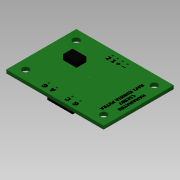
# Autodesk Inventor part: UVTRON
Saved by Autodesk Inventor 2015 SP1 (Build 190203100, 203)
## iProperties
Created: 2015-01-27
Part Number: UVTRON
Material: Generic
Document SubType Name: Modeling
Designer: Rafi Kurnia Putra
Density: 1 g/cm^3
Appearance: Smooth - Dark Forest Green
Mass: 4.62788 g
Surface Area: 45.4293 cm^2
Volume: 4.62788 cm^3
Author: Rafi Kurnia Putra
Autodesk Inventor part; units mm, degrees
ref_plane "YZ Plane" through (0, 0, 0) normal (1, 0, 0) x (0, 1, 0)
ref_plane "XZ Plane" through (0, 0, 0) normal (0, 1, 0) x (-1, 0, 0)
ref_plane "XY Plane" through (0, 0, 0) normal (0, 0, 1) x (1, 0, 0)
sketch "Sketch1" plane through (0, 0, 0) normal (0, 1, 0) x (-1, 0, 0)
  line L0 (25, -18) -> (-25, -18)
  line L1 (-25, -18) -> (-25, 18)
  line L2 (-25, 18) -> (25, 18)
  line L3 (25, 18) -> (25, -18)
  line L4 (25, 0) -> (25, 18)
  line L5 (25, 18) -> (0, 18)
  circle A0 centre (20, 13) radius 1.75
  circle A1 centre (-20, 13) radius 1.75
  circle A2 centre (20, -13) radius 1.75
  circle A3 centre (-20, -13) radius 1.75
  line L6 (0, -18) -> (0, 18) construction
  circle A4 centre (1.27, 15.5) radius 0.5
  circle A5 centre (3.81, 15.5) radius 0.5
  circle A6 centre (-1.27, 15.5) radius 0.5
  circle A7 centre (-3.81, 15.5) radius 0.5
  circle A8 centre (-4, -13) radius 0.5
  circle A9 centre (-8, -13) radius 0.5
  circle A10 centre (4, -13) radius 0.5
  circle A11 centre (8, -13) radius 0.5
  point P0 (0, 0)
  dimension "d0" = 50
  dimension "d1" = 36
  dimension "d10" = 3.5
  dimension "d12" = 5
  dimension "d13" = 5
  dimension "d16" = 1
  dimension "d17" = 1.27
  dimension "d18" = 2.5
  dimension "d19" = 1
  dimension "d20" = 2.54
  dimension "d21" = 1
  dimension "d22" = 4
  dimension "d23" = 1
  dimension "d24" = 4
  dimension "d41" = 12
  dimension "d43" = 40
  dimension "d44" = 26
  constraints: 14 end point, 12 centre point, 4 symmetric about line, 2 horizontal, 2 parallel, 2 perpendicular, 1 midpoint, 1 vertical, 4 other
  measures "d0" distance of L1.end L2.end
  measures "d1" distance of L0.end L1.end
  measures "d10" diameter of A2
  measures "d12" distance from line of A2.centre L0
  measures "d13" distance from line of A2.centre L3
  measures "d16" diameter of A4
  measures "d17" distance from line of L6 A4.centre
  measures "d18" distance from line of L2 A4.centre
  measures "d19" diameter of A5
  measures "d20" distance of A5.centre A4.centre
  measures "d21" diameter of A8
  measures "d22" distance from line of A8.centre L6
  measures "d23" diameter of A9
  measures "d24" distance of A9.centre A8.centre
  measures "d41" distance of A9.centre A3.centre
  measures "d43" distance of A1.centre A0.centre
  measures "d44" distance of A3.centre A1.centre
extrude "Extrusion1" add sketch "Sketch1" along normal mid plane 1.7
sketch "Sketch2" plane through (0, 0.85, 0) normal (0, 1, 0) x (1, 0, 0)
  line L0 (-14.7399, 7.1996) -> (-1.7399, 7.1996)
  line L1 (-1.7399, 7.1996) -> (-1.7399, -5.8004)
  line L2 (-1.7399, -5.8004) -> (-14.7399, -5.8004)
  line L3 (-14.7399, -5.8004) -> (-14.7399, 7.1996)
  point P0 (0, 0)
  dimension "d27" = 13
  dimension "d28" = 13
  constraints: 8 end point, 2 parallel, 1 horizontal, 1 perpendicular
  measures "d27" distance of L1.end L2.end
  measures "d28" distance of L0.end L1.end
extrude "Extrusion2" add sketch "Sketch2" along normal blind 12
sketch "Sketch3" plane through (0, -0.85, 0) normal (0, -1, 0) x (1, 0, 0)
  line L0 (-14.7399, 5.8004) -> (-7.7399, 5.8004)
  line L1 (-7.7399, 5.8004) -> (-7.7399, 0.8004)
  line L2 (-7.7399, 0.8004) -> (-14.7399, 0.8004)
  line L3 (-14.7399, 0.8004) -> (-14.7399, 5.8004)
  point P0 (0, 0)
  dimension "d31" = 7
  dimension "d32" = 5
  constraints: 8 end point, 2 parallel, 1 horizontal, 1 perpendicular
  measures "d31" distance of L1.end L2.end
  measures "d32" distance of L0.end L1.end
extrude "Extrusion3" add sketch "Sketch3" along normal blind 2.5
sketch "Sketch4" plane through (0, 0.85, 0) normal (0, 1, 0) x (1, 0, 0)
  line L0 (-4.7519, -12.75) -> (-3.9944, -12.75) construction
  line L1 (-3.9944, -12.75) -> (-3.9944, -13.9894) construction
  line L2 (-3.9944, -13.9894) -> (-4.7519, -13.9894) construction
  line L3 (-4.7519, -13.9894) -> (-4.7519, -12.75) construction
  line L4 (-2.1513, -12.7634) -> (-1.6525, -12.7634) construction
  line L5 (-1.6525, -12.7634) -> (-1.6525, -14.0027) construction
  line L6 (-1.6525, -14.0027) -> (-2.1513, -14.0027) construction
  line L7 (-2.1513, -14.0027) -> (-2.1513, -12.7634) construction
  line L8 (0.0686, -14.1363) -> (0.0686, -12.897) construction
  line L9 (0.0686, -12.897) -> (0.5673, -12.897) construction
  line L10 (0.5673, -12.897) -> (0.5673, -14.1363) construction
  line L11 (0.5673, -14.1363) -> (0.0686, -14.1363) construction
  line L12 (1.0686, 4.3486) -> (9.004, 4.3486) construction
  line L13 (9.004, 4.3486) -> (9.004, 3.8499) construction
  line L14 (9.004, 3.8499) -> (1.0686, 3.8499) construction
  line L15 (1.0686, 3.8499) -> (1.0686, 4.3486) construction
  line L16 (2.9588, -14.8877) -> (2.9588, -13.6483) construction
  line L17 (2.9588, -13.6483) -> (3.4575, -13.6483) construction
  line L18 (3.4575, -13.6483) -> (3.4575, -14.8877) construction
  line L19 (3.4575, -14.8877) -> (2.9588, -14.8877) construction
  line L20 (-3.0733, 9.8872) -> (-3.8308, 9.8872) construction
  line L21 (-3.8308, 9.8872) -> (-3.8308, 11.1266) construction
  line L22 (-3.8308, 11.1266) -> (-3.0733, 11.1266) construction
  line L23 (-3.0733, 11.1266) -> (-3.0733, 9.8872) construction
  line L24 (4.9547, 10.9292) -> (4.9547, 9.7419) construction
  line L25 (4.9547, 9.7419) -> (4.1972, 9.7419) construction
  line L26 (4.1972, 9.7419) -> (4.1972, 10.9292) construction
  line L27 (4.1972, 10.9292) -> (4.9547, 10.9292) construction
  line L28 (9.0783, 10.888) -> (9.0783, 9.7007) construction
  line L29 (9.0783, 9.7007) -> (8.3208, 9.7007) construction
  line L30 (8.3208, 9.7007) -> (8.3208, 10.888) construction
  line L31 (8.3208, 10.888) -> (9.0783, 10.888) construction
  line L32 (-6.789, 11.003) -> (-6.789, 9.8157) construction
  line L33 (-6.789, 9.8157) -> (-7.5465, 9.8157) construction
  line L34 (-7.5465, 9.8157) -> (-7.5465, 11.003) construction
  line L35 (-7.5465, 11.003) -> (-6.789, 11.003) construction
  point P0 (0, 0)
  point P1 (19.4358, -0.4507)
  constraints: 18 other
sketch "Sketch5" plane through (0, 0.85, 0) normal (0, 1, 0) x (1, 0, 0)
  circle A0 centre (-20, 13) radius 1.75 projected
  circle A1 centre (20, 13) radius 1.75 projected
  circle A2 centre (20, -13) radius 1.75 projected
  circle A3 centre (-20, -13) radius 1.75 projected
  circle A4 centre (-20, 13) radius 2.5
  circle A5 centre (-20, -13) radius 2.5
  circle A6 centre (20, 13) radius 2.5
  circle A7 centre (20, -13) radius 2.5
  point P0 (0, 0)
  dimension "d35" = 5
  dimension "d36" = 5
  dimension "d37" = 5
  dimension "d38" = 5
  constraints: 4 centre point, 4 coincident
  measures "d35" diameter of A4
  measures "d36" diameter of A5
  measures "d37" diameter of A6
  measures "d38" diameter of A7
extrude "Extrusion4" add sketch "Sketch5" along normal blind 0.1
sketch "Sketch6" plane through (0, -0.85, 0) normal (0, -1, 0) x (1, 0, 0)
  line L0 (-3.0976, -15.0106) -> (-3.0976, -16.25) construction
  line L1 (-3.0976, -16.25) -> (-3.8551, -16.25) construction
  line L2 (-3.8551, -16.25) -> (-3.8551, -15.0106) construction
  line L3 (-3.8551, -15.0106) -> (-3.0976, -15.0106) construction
  line L4 (4.9305, -15.208) -> (4.9305, -16.3953) construction
  line L5 (4.9305, -16.3953) -> (4.173, -16.3953) construction
  line L6 (4.173, -16.3953) -> (4.173, -15.208) construction
  line L7 (4.173, -15.208) -> (4.9305, -15.208) construction
  line L8 (9.0541, -15.2492) -> (9.0541, -16.4365) construction
  line L9 (9.0541, -16.4365) -> (8.2966, -16.4365) construction
  line L10 (8.2966, -16.4365) -> (8.2966, -15.2492) construction
  line L11 (8.2966, -15.2492) -> (9.0541, -15.2492) construction
  line L12 (-6.8133, -15.1342) -> (-6.8133, -16.3215) construction
  line L13 (-6.8133, -16.3215) -> (-7.5708, -16.3215) construction
  line L14 (-7.5708, -16.3215) -> (-7.5708, -15.1342) construction
  line L15 (-7.5708, -15.1342) -> (-6.8133, -15.1342) construction
  line L16 (-4.6604, 14.3064) -> (-3.9029, 14.3064) construction
  line L17 (-3.9029, 14.3064) -> (-3.9029, 13.067) construction
  line L18 (-3.9029, 13.067) -> (-4.6604, 13.067) construction
  line L19 (-4.6604, 13.067) -> (-4.6604, 14.3064) construction
  line L20 (-2.0597, 13.0536) -> (-2.0597, 14.293) construction
  line L21 (-2.0597, 14.293) -> (-1.561, 14.293) construction
  line L22 (-1.561, 14.293) -> (-1.561, 13.0536) construction
  line L23 (-1.561, 13.0536) -> (-2.0597, 13.0536) construction
  line L24 (0.1602, 12.92) -> (0.1602, 14.1594) construction
  line L25 (0.1602, 14.1594) -> (0.6589, 14.1594) construction
  line L26 (0.6589, 14.1594) -> (0.6589, 12.92) construction
  line L27 (0.6589, 12.92) -> (0.1602, 12.92) construction
  line L28 (3.0504, 12.1687) -> (3.0504, 13.408) construction
  line L29 (3.0504, 13.408) -> (3.5491, 13.408) construction
  line L30 (3.5491, 13.408) -> (3.5491, 12.1687) construction
  line L31 (3.5491, 12.1687) -> (3.0504, 12.1687) construction
  point P0 (0, 0)
  point P1 (19.4358, -0.4507)
  constraints: 17 other
body "Solid1"
